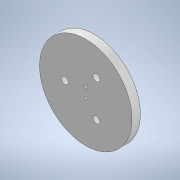
# Autodesk Inventor part: Tractor_Static_2
Saved by Autodesk Inventor 2022 (Build 260153070, 153G)
## iProperties
Created: 2022-03-05
Part Number: Tractor_Static_2
Material: Generic
Document SubType Name: Modeling
Designer: a laptop
Density: 1 g/cm^3
Appearance: Default
Author: a laptop
Autodesk Inventor part; units mm, degrees
ref_plane "YZ Plane" through (0, 0, 0) normal (1, 0, 0) x (0, 1, 0)
ref_plane "XZ Plane" through (0, 0, 0) normal (0, 1, 0) x (-1, 0, 0)
ref_plane "XY Plane" through (0, 0, 0) normal (0, 0, 1) x (1, 0, 0)
sketch "Sketch1" plane through (0, 0, 0) normal (0, 0, 1) x (1, 0, 0)
  circle A0 centre (0, 0) radius 34.925 construction
  circle A1 centre (0, 0) radius 54.75
  circle A2 centre (12.4625, 21.5857) radius 4
  circle A3 centre (-24.925, 0) radius 4
  circle A4 centre (12.4625, -21.5857) radius 4
  line L0 (-24.925, 0) -> (12.4625, 21.5857) construction
  line L1 (12.4625, 21.5857) -> (12.4625, -21.5857) construction
  line L2 (12.4625, -21.5857) -> (-24.925, 0) construction
  line L3 (12.4625, 21.5857) -> (17.4625, 30.2459) construction
  line L4 (12.4625, -21.5857) -> (17.4625, -30.2459) construction
  line L5 (-24.925, 0) -> (-34.925, 0) construction
  circle A5 centre (0, 0) radius 11.075
  dimension "d0" = 69.85
  dimension "d1" = 109.5
  dimension "d2" = 8
  dimension "d3" = 10
  dimension "d4" = 22.15
  constraints: 12 end point, 6 centre point, 4 equal length, 3 coincident, 3 line through centre, 3 point on circle, 2 equal radius, 1 horizontal
  measures "d0" diameter of A0
  measures "d1" diameter of A1
  measures "d2" diameter of A2
  measures "d3" distance of L0.end L3.end
  measures "d4" diameter of A5
extrude "Extrusion1" add sketch "Sketch1" along normal blind 10
body "Solid1"
